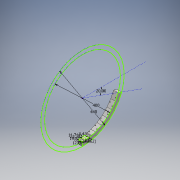
# Autodesk Inventor part: fourche_v2_sans_radiateurs
Saved by Autodesk Inventor 2016 (Build 200138000, 138)
## iProperties
Created: 2018-02-21
Part Number: fourche_v2_sans_radiateurs
Material: Generic
Document SubType Name: Modeling
Designer: mbouhier
Density: 1 g/cm^3
Appearance: Default
Author: mbouhier
Autodesk Inventor part; units mm, degrees
ref_plane "YZ Plane" through (0, 0, 0) normal (1, 0, 0) x (0, 1, 0)
ref_plane "XZ Plane" through (0, 0, 0) normal (0, 1, 0) x (-1, 0, 0)
ref_plane "XY Plane" through (0, 0, 0) normal (0, 0, 1) x (1, 0, 0)
sketch "Sketch1" plane through (0, 0, 0) normal (1, 0, 0) x (0, 1, 0)
  circle A0 centre (0, 0) radius 200 construction
  line L0 (0, 0) -> (293, 0) construction
  line L1 (0, 0) -> (315, -114.6506) construction
  line L2 (0, 0) -> (335.216, 0) construction
  line L3 (0, -200) -> (-34.7296, -196.9616)
  line L4 (-34.7296, -196.9616) -> (-68.404, -187.9385)
  line L5 (-68.404, -187.9385) -> (-100, -173.2051)
  line L6 (-100, -173.2051) -> (-128.5575, -153.2089)
  line L7 (-128.5575, -153.2089) -> (-153.2089, -128.5575)
  line L8 (-153.2089, -128.5575) -> (-173.2051, -100)
  line L9 (-173.2051, -100) -> (-187.9385, -68.404)
  line L10 (-187.9385, -68.404) -> (-196.9616, -34.7296)
  line L11 (-196.9616, -34.7296) -> (-200, 0)
  line L12 (-200, 0) -> (-196.9616, 34.7296)
  line L13 (-196.9616, 34.7296) -> (-187.9385, 68.404)
  line L14 (-187.9385, 68.404) -> (-173.2051, 100)
  line L15 (-173.2051, 100) -> (-153.2089, 128.5575)
  line L16 (-153.2089, 128.5575) -> (-128.5575, 153.2089)
  line L17 (-128.5575, 153.2089) -> (-100, 173.2051)
  line L18 (-100, 173.2051) -> (-68.404, 187.9385)
  line L19 (-68.404, 187.9385) -> (-34.7296, 196.9616)
  line L20 (-34.7296, 196.9616) -> (0, 200)
  line L21 (0, 200) -> (34.7296, 196.9616)
  line L22 (34.7296, 196.9616) -> (68.404, 187.9385)
  line L23 (68.404, 187.9385) -> (100, 173.2051)
  line L24 (100, 173.2051) -> (128.5575, 153.2089)
  line L25 (128.5575, 153.2089) -> (153.2089, 128.5575)
  line L26 (153.2089, 128.5575) -> (173.2051, 100)
  line L27 (173.2051, 100) -> (187.9385, 68.404)
  line L28 (187.9385, 68.404) -> (196.9616, 34.7296)
  line L29 (196.9616, 34.7296) -> (200, 0)
  line L30 (200, 0) -> (196.9616, -34.7296)
  line L31 (196.9616, -34.7296) -> (187.9385, -68.404)
  line L32 (187.9385, -68.404) -> (173.2051, -100)
  line L33 (173.2051, -100) -> (153.2089, -128.5575)
  line L34 (153.2089, -128.5575) -> (128.5575, -153.2089)
  line L35 (128.5575, -153.2089) -> (100, -173.2051)
  line L36 (100, -173.2051) -> (68.404, -187.9385)
  line L37 (68.404, -187.9385) -> (34.7296, -196.9616)
  line L38 (34.7296, -196.9616) -> (0, -200)
  circle A1 centre (0, 0) radius 220 construction
  line L39 (0, -220) -> (-38.2026, -216.6577)
  line L40 (-38.2026, -216.6577) -> (-75.2444, -206.7324)
  line L41 (-75.2444, -206.7324) -> (-110, -190.5256)
  line L42 (-110, -190.5256) -> (-141.4133, -168.5298)
  line L43 (-141.4133, -168.5298) -> (-168.5298, -141.4133)
  line L44 (-168.5298, -141.4133) -> (-190.5256, -110)
  line L45 (-190.5256, -110) -> (-206.7324, -75.2444)
  line L46 (-206.7324, -75.2444) -> (-216.6577, -38.2026)
  line L47 (-216.6577, -38.2026) -> (-220, 0)
  line L48 (-220, 0) -> (-216.6577, 38.2026)
  line L49 (-216.6577, 38.2026) -> (-206.7324, 75.2444)
  line L50 (-206.7324, 75.2444) -> (-190.5256, 110)
  line L51 (-190.5256, 110) -> (-168.5298, 141.4133)
  line L52 (-168.5298, 141.4133) -> (-141.4133, 168.5298)
  line L53 (-141.4133, 168.5298) -> (-110, 190.5256)
  line L54 (-110, 190.5256) -> (-75.2444, 206.7324)
  line L55 (-75.2444, 206.7324) -> (-38.2026, 216.6577)
  line L56 (-38.2026, 216.6577) -> (0, 220)
  line L57 (0, 220) -> (38.2026, 216.6577)
  line L58 (38.2026, 216.6577) -> (75.2444, 206.7324)
  line L59 (75.2444, 206.7324) -> (110, 190.5256)
  line L60 (110, 190.5256) -> (141.4133, 168.5298)
  line L61 (141.4133, 168.5298) -> (168.5298, 141.4133)
  line L62 (168.5298, 141.4133) -> (190.5256, 110)
  line L63 (190.5256, 110) -> (206.7324, 75.2444)
  line L64 (206.7324, 75.2444) -> (216.6577, 38.2026)
  line L65 (216.6577, 38.2026) -> (220, 0)
  line L66 (220, 0) -> (216.6577, -38.2026)
  line L67 (216.6577, -38.2026) -> (206.7324, -75.2444)
  line L68 (206.7324, -75.2444) -> (190.5256, -110)
  line L69 (190.5256, -110) -> (168.5298, -141.4133)
  line L70 (168.5298, -141.4133) -> (141.4133, -168.5298)
  line L71 (141.4133, -168.5298) -> (110, -190.5256)
  line L72 (110, -190.5256) -> (75.2444, -206.7324)
  line L73 (75.2444, -206.7324) -> (38.2026, -216.6577)
  line L74 (38.2026, -216.6577) -> (0, -220)
  line L75 (0, -200) -> (0, -220)
  line L76 (187.9385, -68.404) -> (206.7324, -75.2444)
  dimension "d0" = 400
  dimension "d2" = 440
  dimension "d1" = 20
  constraints: 154 end point, 4 coincident, 2 horizontal, 2 vertical alignment, 1 equal length, 1 vertical, 150 other
  measures "d1" angle of L1 L2
extrude "Extrusion1" add sketch "Sketch1" against normal blind 23 contours L38 L37 L36 L35 L34 L33 L32 L76 L68 L69 L70 L71 L72 L73 L74 L75
sketch "Sketch2" plane through (-23, 34.7296, -196.9616) normal (0, -0.0871557, 0.9961947) x (1, 0, 0)
  line L0 (23, 0) -> (23, -34.8623)
  line L1 (23, 0) -> (0, 0)
  line L2 (0, -34.8623) -> (0, 0)
  line L3 (23, -34.8623) -> (0, -34.8623)
  line L4 (0, -33.9311) -> (23, -33.9311)
  line L5 (23, -33.9311) -> (23, -0.9311)
  line L6 (23, -0.9311) -> (0, -0.9311)
  line L7 (0, -0.9311) -> (0, -33.9311)
  line L8 (0, -33.9311) -> (23, -0.9311) construction
  line L9 (23, -33.9311) -> (0, -0.9311) construction
  point P0 (23, -17.4311)
  point P1 (11.5, -17.4311)
  point P2 (3.4356, -12.6296)
  point P3 (19.8273, -22.2197)
  dimension "d5" = 34.8623
  dimension "d6" = 23
  dimension "d7" = 23
  dimension "d8" = 33
  dimension "d10" = 3.4356
  dimension "d11" = 21.3015
  dimension "d12" = 19.8273
  dimension "d13" = 11.7114
  constraints: 20 end point, 2 collinear, 2 midpoint, 2 parallel, 1 horizontal, 1 perpendicular
  measures "d5" distance of L0.start L0.end
  measures "d6" distance of L0.end L2.start
  measures "d7" distance of L6.end L5.end
  measures "d8" distance of L5.end L4.end
  measures "d10" distance from line of point (3.436, -12.63) L2
  measures "d11" distance from line of point (3.436, -12.63) L4
  measures "d12" distance from line of point (19.827, -22.22) L2
  measures "d13" distance from line of point (19.827, -22.22) L4
sketch "Sketch9" plane through (-23.1315, 68.3978, -187.9402) normal (0, -0.258819, 0.9659258) x (1, 0, 0)
  line L0 (23, 0) -> (23, -34.8623)
  line L1 (23, 0) -> (0, 0)
  line L2 (0, -34.8623) -> (0, 0)
  line L3 (23, -34.8623) -> (0, -34.8623)
  line L4 (0, -33.9311) -> (23, -33.9311)
  line L5 (23, -33.9311) -> (23, -0.9311)
  line L6 (23, -0.9311) -> (0, -0.9311)
  line L7 (0, -0.9311) -> (0, -33.9311)
  line L8 (0, -33.9311) -> (23, -0.9311) construction
  line L9 (23, -33.9311) -> (0, -0.9311) construction
  point P0 (23, -17.4311)
  point P1 (11.5, -17.4311)
  point P2 (3.4356, -12.6296)
  point P3 (19.8273, -22.2197)
  dimension "d124" = 34.8623
  dimension "d125" = 23
  dimension "d116" = 23
  dimension "d117" = 33
  dimension "d115" = 3.4356
  dimension "d114" = 21.3015
  dimension "d113" = 19.8273
  dimension "d112" = 11.7114
  constraints: 20 end point, 2 collinear, 2 midpoint, 2 parallel, 1 horizontal, 1 perpendicular
  measures "d124" distance of L0.start L0.end
  measures "d125" distance of L0.end L2.start
  measures "d116" distance of L6.end L5.end
  measures "d117" distance of L5.end L4.end
  measures "d115" distance from line of point (3.436, -12.63) L2
  measures "d114" distance from line of point (3.436, -12.63) L4
  measures "d113" distance from line of point (19.827, -22.22) L2
  measures "d112" distance from line of point (19.827, -22.22) L4
hole "Hole8" at (-19.6959, 56.1985, -191.209) at (-3.3042, 46.9352, -193.6911) direction (0, 0.258819, -0.9659258) diameter 4 depth 6
sketch "Sketch10" plane through (-23.1315, 99.9942, -173.2078) normal (0, -0.4226183, 0.9063078) x (1, 0, 0)
  line L0 (23, 0) -> (23, -34.8623)
  line L1 (23, 0) -> (0, 0)
  line L2 (0, -34.8623) -> (0, 0)
  line L3 (23, -34.8623) -> (0, -34.8623)
  line L4 (0, -33.9311) -> (23, -33.9311)
  line L5 (23, -33.9311) -> (23, -0.9311)
  line L6 (23, -0.9311) -> (0, -0.9311)
  line L7 (0, -0.9311) -> (0, -33.9311)
  line L8 (0, -33.9311) -> (23, -0.9311) construction
  line L9 (23, -33.9311) -> (0, -0.9311) construction
  point P0 (23, -17.4311)
  point P1 (11.5, -17.4311)
  point P2 (3.4356, -12.6296)
  point P3 (19.8273, -22.2197)
  dimension "d139" = 34.8623
  dimension "d140" = 23
  dimension "d131" = 23
  dimension "d132" = 33
  dimension "d130" = 3.4356
  dimension "d129" = 21.3015
  dimension "d128" = 19.8273
  dimension "d127" = 11.7114
  constraints: 20 end point, 2 collinear, 2 midpoint, 2 parallel, 1 horizontal, 1 perpendicular
  measures "d139" distance of L0.start L0.end
  measures "d140" distance of L0.end L2.start
  measures "d131" distance of L6.end L5.end
  measures "d132" distance of L5.end L4.end
  measures "d130" distance from line of point (3.436, -12.63) L2
  measures "d129" distance from line of point (3.436, -12.63) L4
  measures "d128" distance from line of point (19.827, -22.22) L2
  measures "d127" distance from line of point (19.827, -22.22) L4
hole "Hole9" at (-19.6959, 88.5478, -178.5453) at (-3.3042, 79.8562, -182.5983) direction (0, 0.4226183, -0.9063078) diameter 4 depth 6
sketch "Sketch11" plane through (-23.1315, 128.5522, -153.2126) normal (0, -0.5735764, 0.819152) x (1, 0, 0)
  line L0 (23, 0) -> (23, -34.8623)
  line L1 (23, 0) -> (0, 0)
  line L2 (0, -34.8623) -> (0, 0)
  line L3 (23, -34.8623) -> (0, -34.8623)
  line L4 (0, -33.9311) -> (23, -33.9311)
  line L5 (23, -33.9311) -> (23, -0.9311)
  line L6 (23, -0.9311) -> (0, -0.9311)
  line L7 (0, -0.9311) -> (0, -33.9311)
  line L8 (0, -33.9311) -> (23, -0.9311) construction
  line L9 (23, -33.9311) -> (0, -0.9311) construction
  point P0 (23, -17.4311)
  point P1 (11.5, -17.4311)
  point P2 (3.4356, -12.6296)
  point P3 (19.8273, -22.2197)
  dimension "d154" = 34.8623
  dimension "d155" = 23
  dimension "d146" = 23
  dimension "d147" = 33
  dimension "d145" = 3.4356
  dimension "d144" = 21.3015
  dimension "d143" = 19.8273
  dimension "d142" = 11.7114
  constraints: 20 end point, 2 collinear, 2 midpoint, 2 parallel, 1 horizontal, 1 perpendicular
  measures "d154" distance of L0.start L0.end
  measures "d155" distance of L0.end L2.start
  measures "d146" distance of L6.end L5.end
  measures "d147" distance of L5.end L4.end
  measures "d145" distance from line of point (3.436, -12.63) L2
  measures "d144" distance from line of point (3.436, -12.63) L4
  measures "d143" distance from line of point (19.827, -22.22) L2
  measures "d142" distance from line of point (19.827, -22.22) L4
hole "Hole10" at (-19.6959, 118.2066, -160.4567) at (-3.3042, 110.3509, -165.9573) direction (0, 0.5735764, -0.819152) diameter 4 depth 6
sketch "Sketch12" plane through (-23.1315, 153.2043, -128.5621) normal (0, -0.7071068, 0.7071068) x (1, 0, 0)
  line L0 (23, 0) -> (23, -34.8623)
  line L1 (23, 0) -> (0, 0)
  line L2 (0, -34.8623) -> (0, 0)
  line L3 (23, -34.8623) -> (0, -34.8623)
  line L4 (0, -33.9311) -> (23, -33.9311)
  line L5 (23, -33.9311) -> (23, -0.9311)
  line L6 (23, -0.9311) -> (0, -0.9311)
  line L7 (0, -0.9311) -> (0, -33.9311)
  line L8 (0, -33.9311) -> (23, -0.9311) construction
  line L9 (23, -33.9311) -> (0, -0.9311) construction
  point P0 (23, -17.4311)
  point P1 (11.5, -17.4311)
  point P2 (3.4356, -12.6296)
  point P3 (19.8273, -22.2197)
  dimension "d169" = 34.8623
  dimension "d170" = 23
  dimension "d161" = 23
  dimension "d162" = 33
  dimension "d160" = 3.4356
  dimension "d159" = 21.3015
  dimension "d158" = 19.8273
  dimension "d157" = 11.7114
  constraints: 20 end point, 2 collinear, 2 midpoint, 2 parallel, 1 horizontal, 1 perpendicular
  measures "d169" distance of L0.start L0.end
  measures "d170" distance of L0.end L2.start
  measures "d161" distance of L6.end L5.end
  measures "d162" distance of L5.end L4.end
  measures "d160" distance from line of point (3.436, -12.63) L2
  measures "d159" distance from line of point (3.436, -12.63) L4
  measures "d158" distance from line of point (19.827, -22.22) L2
  measures "d157" distance from line of point (19.827, -22.22) L4
hole "Hole11" at (-19.6959, 144.2738, -137.4926) at (-3.3042, 137.4926, -144.2738) direction (0, 0.7071068, -0.7071068) diameter 4 depth 6
sketch "Sketch13" plane through (-23.1315, 173.2014, -100.0053) normal (0, -0.819152, 0.5735764) x (1, 0, 0)
  line L0 (23, 0) -> (23, -34.8623)
  line L1 (23, 0) -> (0, 0)
  line L2 (0, -34.8623) -> (0, 0)
  line L3 (23, -34.8623) -> (0, -34.8623)
  line L4 (0, -33.9311) -> (23, -33.9311)
  line L5 (23, -33.9311) -> (23, -0.9311)
  line L6 (23, -0.9311) -> (0, -0.9311)
  line L7 (0, -0.9311) -> (0, -33.9311)
  line L8 (0, -33.9311) -> (23, -0.9311) construction
  line L9 (23, -33.9311) -> (0, -0.9311) construction
  point P0 (23, -17.4311)
  point P1 (11.5, -17.4311)
  point P2 (3.4356, -12.6296)
  point P3 (19.8273, -22.2197)
  dimension "d184" = 34.8623
  dimension "d185" = 23
  dimension "d176" = 23
  dimension "d177" = 33
  dimension "d175" = 3.4356
  dimension "d174" = 21.3015
  dimension "d173" = 19.8273
  dimension "d172" = 11.7114
  constraints: 20 end point, 2 collinear, 2 midpoint, 2 parallel, 1 horizontal, 1 perpendicular
  measures "d184" distance of L0.start L0.end
  measures "d185" distance of L0.end L2.start
  measures "d176" distance of L6.end L5.end
  measures "d177" distance of L5.end L4.end
  measures "d175" distance from line of point (3.436, -12.63) L2
  measures "d174" distance from line of point (3.436, -12.63) L4
  measures "d173" distance from line of point (19.827, -22.22) L2
  measures "d172" distance from line of point (19.827, -22.22) L4
hole "Hole12" at (-19.6959, 165.9573, -110.3509) at (-3.3042, 160.4567, -118.2066) direction (0, 0.819152, -0.5735764) diameter 4 depth 6
sketch "Sketch14" plane through (-23.1315, 187.9358, -68.4099) normal (0, -0.9063078, 0.4226183) x (1, 0, 0)
  line L0 (23, 0) -> (23, -34.8623)
  line L1 (23, 0) -> (0, 0)
  line L2 (0, -34.8623) -> (0, 0)
  line L3 (23, -34.8623) -> (0, -34.8623)
  line L4 (0, -33.9311) -> (23, -33.9311)
  line L5 (23, -33.9311) -> (23, -0.9311)
  line L6 (23, -0.9311) -> (0, -0.9311)
  line L7 (0, -0.9311) -> (0, -33.9311)
  line L8 (0, -33.9311) -> (23, -0.9311) construction
  line L9 (23, -33.9311) -> (0, -0.9311) construction
  point P0 (23, -17.4311)
  point P1 (11.5, -17.4311)
  point P2 (3.4356, -12.6296)
  point P3 (19.8273, -22.2197)
  dimension "d199" = 34.8623
  dimension "d200" = 23
  dimension "d191" = 23
  dimension "d192" = 33
  dimension "d190" = 3.4356
  dimension "d189" = 21.3015
  dimension "d188" = 19.8273
  dimension "d187" = 11.7114
  constraints: 20 end point, 2 collinear, 2 midpoint, 2 parallel, 1 horizontal, 1 perpendicular
  measures "d199" distance of L0.start L0.end
  measures "d200" distance of L0.end L2.start
  measures "d191" distance of L6.end L5.end
  measures "d192" distance of L5.end L4.end
  measures "d190" distance from line of point (3.436, -12.63) L2
  measures "d189" distance from line of point (3.436, -12.63) L4
  measures "d188" distance from line of point (19.827, -22.22) L2
  measures "d187" distance from line of point (19.827, -22.22) L4
hole "Hole13" at (-19.6959, 182.5983, -79.8562) at (-3.3042, 178.5453, -88.5478) direction (0, 0.9063078, -0.4226183) diameter 4 depth 6
sketch "Sketch15" plane through (0, 0, -220) normal (0, -1, 0) x (1, 0, 0)
  line L0 (0, 20) -> (0, 0) projected
  line L1 (0, 20) -> (-23, 20) projected
  line L2 (-23, 0) -> (-23, 20) projected
  line L3 (0, 0) -> (-23, 0) projected
  point P0 (0, 220)
  point P1 (-3, 10)
  point P2 (-20, 10)
  dimension "d201" = 3
  dimension "d202" = 3
  measures "d201" distance from line of L0 point (-3, 10)
  measures "d202" distance from line of L2 point (-20, 10)
hole "Hole14" at (-20, 0, -210) at (-3, 0, -210) direction (0, 1, 0) diameter 4 depth 6 tip angle 118
equation "\"d116\" = d7"
equation "\"d117\" = d8"
equation "\"d115\" = d10"
equation "\"d114\" = d11"
equation "\"d113\" = d12"
equation "\"d112\" = d13"
equation "\"d123\" = d14"
equation "\"d122\" = d19"
equation "\"d131\" = d7"
equation "\"d132\" = d8"
equation "\"d130\" = d10"
equation "\"d129\" = d11"
equation "\"d128\" = d12"
equation "\"d127\" = d13"
equation "\"d138\" = d14"
equation "\"d137\" = d19"
equation "\"d146\" = d7"
equation "\"d147\" = d8"
equation "\"d145\" = d10"
equation "\"d144\" = d11"
equation "\"d143\" = d12"
equation "\"d142\" = d13"
equation "\"d153\" = d14"
equation "\"d152\" = d19"
equation "\"d161\" = d7"
equation "\"d162\" = d8"
equation "\"d160\" = d10"
equation "\"d159\" = d11"
equation "\"d158\" = d12"
equation "\"d157\" = d13"
equation "\"d168\" = d14"
equation "\"d167\" = d19"
equation "\"d176\" = d7"
equation "\"d177\" = d8"
equation "\"d175\" = d10"
equation "\"d174\" = d11"
equation "\"d173\" = d12"
equation "\"d172\" = d13"
equation "\"d183\" = d14"
equation "\"d182\" = d19"
equation "\"d191\" = d7"
equation "\"d192\" = d8"
equation "\"d190\" = d10"
equation "\"d189\" = d11"
equation "\"d188\" = d12"
equation "\"d187\" = d13"
equation "\"d198\" = d14"
equation "\"d197\" = d19"
equation "\"d202\" = d201"
equation "\"d14\" = 4"
equation "\"d19\" = 6"
body "Solid1"
